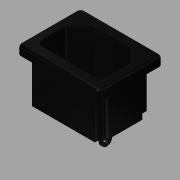
# Autodesk Inventor part: 701W-X202
Saved by Autodesk Inventor 2013 (Build 170138000, 138)
## iProperties
Created: 2014-06-07
Part Number: 701W-X202
Material: Generic
Document SubType Name: Modeling
Designer: Brad
Density: 1 g/cm^3
Author: Brad
Autodesk Inventor part; units mm, degrees
ref_plane "YZ Plane" through (0, 0, 0) normal (1, 0, 0) x (0, 1, 0)
ref_plane "XZ Plane" through (0, 0, 0) normal (0, 1, 0) x (-1, 0, 0)
ref_plane "XY Plane" through (0, 0, 0) normal (0, 0, 1) x (1, 0, 0)
sketch "Sketch1" plane through (0, 0, 0) normal (0, 0, 1) x (1, 0, 0)
  line L0 (-15.35, 11.85) -> (15.35, 11.85)
  line L1 (15.35, 11.85) -> (15.35, -11.85)
  line L2 (15.35, -11.85) -> (-15.35, -11.85)
  line L3 (-15.35, -11.85) -> (-15.35, 11.85)
  point P0 (0, 0)
  dimension "d0" = 30.7
  dimension "d2" = 23.7
  dimension "d3" = 15.35
  dimension "d4" = 11.85
  constraints: 8 end point, 2 parallel, 1 horizontal, 1 perpendicular
  measures "d0" distance of L0.start L0.end
  measures "d2" distance of L0.end L1.end
  measures "d3" distance from line of point (0, 0) L1
  measures "d4" distance from line of point (0, 0) L0
extrude "Extrusion1" add sketch "Sketch1" against normal blind 3.2
sketch "Sketch2" plane through (0, 0, -3.2) normal (0, 0, -1) x (-1, 0, 0)
  line L0 (15.35, -11.85) -> (15.35, 11.85) projected
  line L1 (-11.25, 9.9) -> (11.25, 9.9)
  line L2 (13.25, 6.2453) -> (13.25, -5.9)
  line L3 (11.75, -9.9) -> (-11.75, -9.9)
  line L4 (-13.25, -5.9) -> (-13.25, 6.2453)
  line L5 (11.75, -9.9) -> (11.75, -9.0225)
  arc A0 (11.75, -9.0225) -> (13.25, -5.9) centre (9.25, -5.9) ccw
  line L6 (0, 0) -> (0, 2.1839)
  line L7 (-11.75, -9.9) -> (-11.75, -9.0225)
  arc A1 (-13.25, -5.9) -> (-11.75, -9.0225) centre (-9.25, -5.9) ccw
  line L8 (11.25, 9.9) -> (11.25, 7.4)
  line L9 (11.25, 7.4) -> (13.25, 6.2453)
  line L10 (-11.25, 9.9) -> (-11.25, 7.4)
  line L11 (-11.25, 7.4) -> (-13.25, 6.2453)
  dimension "d10" = 9.9
  dimension "d11" = 13.25
  dimension "d13" = 8
  dimension "d15" = 1.5
  dimension "d19" = 120
  dimension "d20" = 19.8
  dimension "d21" = 2
  dimension "d22" = 2.5
  constraints: 22 end point, 7 symmetric about line, 5 parallel, 4 point on circle, 2 centre point, 2 perpendicular, 2 tangent, 1 other
  measures "d10" distance from line of L6.start L3
  measures "d11" distance from line of L6.start L2
  measures "d13" diameter of A0
  measures "d15" distance between parallel lines of L2 L5
  measures "d19" angle of L9 L8
  measures "d20" distance between parallel lines of L3 L1
  measures "d21" distance between parallel lines of L2 L8
  measures "d22" distance of L1.end L8.end
extrude "Extrusion2" add sketch "Sketch2" along normal blind 16
sketch "Sketch3" plane through (0, 0, -19.2) normal (0, 0, -1) x (-1, 0, 0)
  line L0 (-11.25, 9.9) -> (-11.25, 7.4) projected
  line L1 (-1.75, 7.5) -> (-1.75, -0.5)
  line L2 (-1.75, -0.5) -> (1.75, -0.5)
  line L3 (1.75, -0.5) -> (1.75, 7.5)
  line L4 (1.75, 7.5) -> (-1.75, 7.5)
  line L5 (-9.5, 2) -> (-9.5, -6)
  line L6 (-9.5, -6) -> (-6, -6)
  line L7 (-6, -6) -> (-6, 2)
  line L8 (-6, 2) -> (-9.5, 2)
  line L9 (6, 2) -> (6, -6)
  line L10 (6, -6) -> (9.5, -6)
  line L11 (9.5, -6) -> (9.5, 2)
  line L12 (9.5, 2) -> (6, 2)
  point P0 (0, 0)
  dimension "d25" = 3.5
  dimension "d27" = 8
  dimension "d28" = 1.75
  dimension "d29" = 7.5
  dimension "d30" = 3.5
  dimension "d31" = 8
  dimension "d32" = 3.5
  dimension "d33" = 8
  dimension "d34" = 2
  dimension "d35" = 2
  dimension "d36" = 6
  dimension "d37" = 6
  constraints: 24 end point, 7 parallel, 3 perpendicular
  measures "d25" distance of L1.end L2.end
  measures "d27" distance of L2.end L3.end
  measures "d28" distance from line of point (0, 0) L3
  measures "d29" distance from line of point (0, 0) L4
  measures "d30" distance of L5.end L7.start
  measures "d31" distance of L7.start L8.start
  measures "d32" distance of L9.end L11.start
  measures "d33" distance of L11.start L12.start
  measures "d34" distance from line of point (0, 0) L8
  measures "d35" distance from line of point (0, 0) L12
  measures "d36" distance from line of point (0, 0) L9
  measures "d37" distance from line of point (0, 0) L7
extrude "Extrusion3" add sketch "Sketch3" along normal blind 1.5
sketch "Sketch4" plane through (0, 0, -20.7) normal (0, 0, -1) x (-1, 0, 0)
  line L0 (-6, -6) -> (-6, 2) projected
  line L1 (-6, 2) -> (-9.5, 2) projected
  line L2 (-8.25, 0) -> (-8.25, -4)
  line L3 (-8.25, -4) -> (-7.25, -4)
  line L4 (-7.25, -4) -> (-7.25, 0)
  line L5 (-7.25, 0) -> (-8.25, 0)
  point P0 (-9.5, -6)
  point P1 (0, 0)
  dimension "d40" = 4
  dimension "d42" = 1
  dimension "d43" = 1.25
  dimension "d44" = 3.5
  dimension "d45" = 8
  dimension "d46" = 2
  constraints: 8 end point, 2 parallel, 2 perpendicular
  measures "d40" distance of L2.start L2.end
  measures "d42" distance of L2.end L3.end
  measures "d43" distance between parallel lines of L0 L4
  measures "d44" distance of point (-9.5, -6) L0.start
  measures "d45" distance of L0.start L0.end
  measures "d46" distance between parallel lines of L1 L5
extrude "Extrusion4" add sketch "Sketch4" along normal blind 5.5
sketch "Sketch6" plane through (0, 0, -20.7) normal (0, 0, -1) x (-1, 0, 0)
  line L0 (-1.75, -0.5) -> (1.75, -0.5) projected
  line L1 (1.75, -0.5) -> (1.75, 7.5) projected
  line L2 (1.75, 7.5) -> (-1.75, 7.5) projected
  line L3 (-0.5, 5.5) -> (0.5, 5.5)
  line L4 (0.5, 5.5) -> (0.5, 1.5)
  line L5 (0.5, 1.5) -> (-0.5, 1.5)
  line L6 (-0.5, 1.5) -> (-0.5, 5.5)
  point P0 (0, 0)
  dimension "d55" = 1
  dimension "d57" = 4
  dimension "d58" = 1.25
  dimension "d59" = 2
  dimension "d60" = 8
  dimension "d61" = 2
  constraints: 8 end point, 2 parallel, 1 horizontal, 1 perpendicular
  measures "d55" distance of L3.start L3.end
  measures "d57" distance of L3.end L4.end
  measures "d58" distance between parallel lines of L1 L4
  measures "d59" distance between parallel lines of L2 L3
  measures "d60" distance of L0.end L1.end
  measures "d61" distance between parallel lines of L0 L5
extrude "Extrusion5" add sketch "Sketch6" along normal blind 5.5
sketch "Sketch7" plane through (0, 0, -20.7) normal (0, 0, -1) x (-1, 0, 0)
  line L0 (9.5, -6) -> (9.5, 2) projected
  line L1 (9.5, 2) -> (6, 2) projected
  line L2 (8.25, -4) -> (7.25, -4)
  line L3 (7.25, -4) -> (7.25, 0)
  line L4 (7.25, 0) -> (8.25, 0)
  line L5 (8.25, 0) -> (8.25, -4)
  point P0 (0, 0)
  dimension "d64" = 2
  dimension "d65" = 4
  dimension "d66" = 1.25
  dimension "d67" = 1
  constraints: 8 end point, 2 parallel, 1 horizontal, 1 perpendicular
  measures "d64" distance between parallel lines of L1 L4
  measures "d65" distance of L4.end L2.start
  measures "d66" distance between parallel lines of L0 L5
  measures "d67" distance of L2.start L2.end
extrude "Extrusion6" add sketch "Sketch7" along normal blind 5.5
sketch "Sketch8" plane through (8.25, -4, -20.7) normal (1, 0, 0) x (0, 0, -1)
  line L0 (0, 0) -> (0, 4) projected
  line L1 (0, 0) -> (5.5, 0) projected
  line L2 (5.5, 4) -> (5.5, 0) projected
  line L3 (0, 4) -> (5.5, 4) projected
  arc A0 (3.5, 0) -> (3.5, 4) centre (3.5, 2) ccw
  arc A1 (3.5, 0.9) -> (3.5, 3.1) centre (3.5, 2) ccw
  line L4 (3.5, 2) -> (2.8, 2)
  arc A2 (2.8, 3.1) -> (2.8, 0.9) centre (2.8, 2) ccw
  line L5 (2.8, 3.1) -> (3.5, 3.1)
  line L6 (3.5, 0.9) -> (2.8, 0.9)
  line L7 (3.5, 4) -> (5.5, 4)
  line L8 (5.5, 4) -> (5.5, 0)
  line L9 (5.5, 0) -> (3.5, 0)
  point P0 (-20.7, 4)
  dimension "d70" = 4
  dimension "d72" = 2.2
  dimension "d73" = 0.7
  dimension "d74" = 2.2
  constraints: 12 end point, 6 point on circle, 5 tangent, 4 parallel, 3 centre point, 2 coincident, 2 point on line, 1 collinear, 1 perpendicular
  measures "d70" diameter of A0
  measures "d72" diameter of A1
  measures "d73" distance of L4.start L4.end
  measures "d74" diameter of A2
extrude "Extrusion7" cut sketch "Sketch8" against normal blind 1 contours A0 L2 L1 | L3 L2 A0 | L6 A2 L5 A1
sketch "Sketch11" plane through (0.5, 1.5, -20.7) normal (1, 0, 0) x (0, 0, -1)
  line L0 (0, 0) -> (0, 4) projected
  line L1 (0, 0) -> (5.5, 0) projected
  line L2 (5.5, 4) -> (5.5, 0) projected
  line L3 (0, 4) -> (5.5, 4) projected
  arc A0 (3.5, 0) -> (3.5, 4) centre (3.5, 2) ccw
  line L4 (3.5, 0) -> (5.5, 0)
  line L5 (5.5, 4) -> (5.5, 0)
  line L6 (5.5, 4) -> (3.5, 4)
  arc A1 (3.5, 0.9) -> (3.5, 3.1) centre (3.5, 2) ccw
  line L7 (3.5, 2) -> (2.8, 2)
  arc A2 (2.8, 3.1) -> (2.8, 0.9) centre (2.8, 2) ccw
  line L8 (2.8, 3.1) -> (3.5, 3.1)
  line L9 (3.5, 0.9) -> (2.8, 0.9)
  point P0 (-20.7, -1.5)
  dimension "d88" = 4
  dimension "d91" = 2.2
  dimension "d92" = 0.7
  dimension "d93" = 2.2
  constraints: 12 end point, 6 point on circle, 5 tangent, 3 centre point, 3 parallel, 2 coincident, 2 point on line, 1 perpendicular
  measures "d88" diameter of A0
  measures "d91" diameter of A1
  measures "d92" distance of L7.start L7.end
  measures "d93" diameter of A2
sketch "Sketch12" plane through (-7.25, -4, -20.7) normal (1, 0, 0) x (0, 0, -1)
  arc A0 (3.5, 0) -> (3.5, 4) centre (3.5, 2) ccw
  arc A1 (3.5, 0.9) -> (3.5, 3.1) centre (3.5, 2) ccw
  line L0 (3.5, 2) -> (2.8, 2)
  arc A2 (2.8, 3.1) -> (2.8, 0.9) centre (2.8, 2) ccw
  line L1 (2.8, 3.1) -> (3.5, 3.1)
  line L2 (3.5, 0.9) -> (2.8, 0.9)
  line L3 (0, 4) -> (5.5, 4) projected
  line L4 (5.5, 4) -> (5.5, 0)
  line L5 (5.5, 4) -> (3.5, 4)
  line L6 (3.5, 0) -> (5.5, 0)
  point P0 (-20.7, -1.5)
  dimension "d94" = 4
  dimension "d95" = 2.2
  dimension "d96" = 0.7
  dimension "d97" = 2.2
  constraints: 12 end point, 7 tangent, 6 point on circle, 3 centre point, 2 coincident, 1 collinear, 1 parallel, 1 perpendicular
  measures "d94" diameter of A0
  measures "d95" diameter of A1
  measures "d96" distance of L0.start L0.end
  measures "d97" diameter of A2
extrude "Extrusion8" cut sketch "Sketch11" against normal blind 1 contours A0 L2 L1 | L3 L2 A0 | L9 A2 L8 A1
extrude "Extrusion9" cut sketch "Sketch12" against normal blind 1 contours L2 A2 L1 A1
sketch "Sketch13" plane through (-7.25, -4, -20.7) normal (1, 0, 0) x (0, 0, -1)
  line L0 (0, 0) -> (5.5, 0) projected
  line L1 (5.5, 4) -> (5.5, 0) projected
  line L2 (0, 4) -> (5.5, 4) projected
  circle A0 centre (3.5, 2) radius 2
  line L3 (3.5, 4) -> (5.5, 4)
  line L4 (5.5, 0) -> (5.5, 4)
  line L5 (3.5, 0) -> (5.5, 0)
  point P0 (-20.7, 4)
  dimension "d102" = 4
  constraints: 6 end point, 3 tangent, 2 perpendicular, 2 point on circle, 2 point on line, 1 centre point, 1 collinear
  measures "d102" diameter of A0
extrude "Extrusion10" cut sketch "Sketch13" against normal blind 1 contours A0 L1 L0 | L2 L1 A0
sketch "Sketch14" plane through (0, 0, 0) normal (0, 0, 1) x (1, 0, 0)
  line L0 (12, -8) -> (-12, -8)
  line L1 (-7, 8) -> (7, 8)
  line L2 (12, 3) -> (12, -8)
  line L3 (7, 8) -> (12, 3)
  line L4 (0, 0) -> (0, 4.7583)
  line L5 (-7, 8) -> (-12, 3)
  line L6 (-12, -8) -> (-12, 3)
  dimension "d107" = 16
  dimension "d108" = 12
  dimension "d109" = 8
  dimension "d110" = 45
  dimension "d111" = 5
  constraints: 14 end point, 3 parallel, 2 symmetric about line, 1 horizontal
  measures "d107" distance between parallel lines of L0 L1
  measures "d108" distance from line of L4.start L2
  measures "d109" distance from line of L4.start L0
  measures "d110" angle of L1 L3
  measures "d111" distance from line of L1.end L2
extrude "Extrusion11" cut sketch "Sketch14" against normal blind 16
fillet "Fillet1" radius 1.5 4 edges at (-15.35, 11.85, -1.6) (15.35, 11.85, -1.6) (15.35, -11.85, -1.6) (-15.35, -11.85, -1.6)
fillet "Fillet2" radius 2 2 edges at (-12, -8, -8) (12, -8, -8)
fillet "Fillet3" radius 1.5 4 edges at (-12, 3, -8) (-7, 8, -8) (7, 8, -8) (12, 3, -8)
fillet "Fillet4" radius 1 8 edges at (-14.9107, 11.4107, 0) (0, 11.85, 0) (14.9107, 11.4107, 0) (15.35, 0, 0) (14.9107, -11.4107, 0) (0, -11.85, 0) (-14.9107, -11.4107, 0) (-15.35, 0, 0)
body "Solid1"
